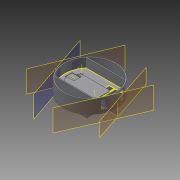
# Autodesk Inventor part: base
Saved by Autodesk Inventor 2014 (Build 180170000, 170)
## iProperties
Created: 2013-06-26
Part Number: base
Material: Generisch
Document SubType Name: Modeling
Designer: hanse
Density: 1 g/cm^3
Appearance: Vorgabe
Author: hanse
Autodesk Inventor part; units mm, degrees
ref_plane "YZ Plane" through (0, 0, 0) normal (1, 0, 0) x (0, 1, 0)
ref_plane "XZ Plane" through (0, 0, 0) normal (0, 1, 0) x (-1, 0, 0)
ref_plane "XY Plane" through (0, 0, 0) normal (0, 0, 1) x (1, 0, 0)
sketch "Skizze1" plane through (0, 0, 0) normal (0, 0, 1) x (1, 0, 0)
  line L0 (29, -20.75) -> (-29, -20.75) projected
  line L1 (29, 20.75) -> (29, -20.75) projected
  line L2 (-29, 20.75) -> (29, 20.75) projected
  line L3 (-29, -20.75) -> (-29, 20.75) projected
  line L4 (4, 34.75) -> (14, 34.75) projected
  line L5 (40.5, 34.75) -> (14, 34.75) projected
  line L6 (14, -34.75) -> (40.5, -34.75) projected
  line L7 (14, -34.75) -> (4, -34.75) projected
  line L8 (40.5, -34.75) -> (40.5, -21.05) projected
  line L9 (40.5, -21.05) -> (40.5, -7.75) projected
  line L10 (40.5, 21.05) -> (40.5, 7.75) projected
  line L11 (40.5, 34.75) -> (40.5, 21.05) projected
  line L12 (4, 34.75) -> (4, 21.05)
  line L13 (4, -34.75) -> (4, -21.05)
  line L14 (13.5, 17.844) -> (13.5, 38.186)
  line L15 (13.5, -17.844) -> (13.5, -38.186)
  line L16 (0, 0) -> (29, 0)
  line L17 (13.5, 17.844) -> (13.5, -17.844)
  line L18 (-15.5, 46.05) -> (42.5, 46.05) projected
  line L19 (42.5, 38.05) -> (-15.5, 38.05) projected
  line L20 (-15.5, -38.05) -> (42.5, -38.05) projected
  line L21 (42.5, -46.05) -> (-15.5, -46.05) projected
  circle A0 centre (12.6975, 0) radius 58.0715
  line L22 (40.5, -7.75) -> (29, -7.75)
  line L23 (29, -7.75) -> (29, -26.5586)
  line L24 (29, -26.5586) -> (40.5, -26.5586)
  line L25 (40.5, -26.5586) -> (40.5, -7.75)
  line L26 (40.5, 7.75) -> (40.5, 26.6995)
  line L27 (40.5, 26.6995) -> (29, 26.6995)
  line L28 (29, 26.6995) -> (29, 7.75)
  line L29 (40.5, 7.75) -> (38.25, 7.75) projected
  line L30 (38.25, 7.75) -> (31.25, 7.75) projected
  line L31 (31.25, 7.75) -> (29, 7.75) projected
  line L32 (40.5, 7.75) -> (29, 7.75)
  line L33 (-32.2663, 36.75) -> (57.6613, 36.75)
  line L34 (-32.2663, -36.75) -> (57.6613, -36.75)
  line L35 (66.1683, 16.4065) -> (68.2, 17.0815)
  dimension "d0" = 2
  dimension "d1" = 2
  constraints: 34 end point, 5 parallel, 5 point on circle, 4 point on line, 4 vertical, 3 collinear, 2 perpendicular, 1 centre point, 1 horizontal, 1 midpoint, 6 other
  measures "d0" distance between parallel lines of L5 L33
  measures "d1" distance between parallel lines of L6 L34
ref_plane "Arbeitsebene1" through (30, 21.05, 2.35) normal (0, 0, 1) x (1, 0, 0)
extrude "Extrusion1" add sketch "Skizze1" along normal up to surface (2.35 mm away) contours L23 L24 L8 L6 L7 L15 L0 | L0 L15 L17 L16 L1 | L15 L34 A0 L33 L14 L2 L3 L0 | L0 L3 L2 L14 L17 L15 | L1 L31 L30 L29 L10 L11 L5 L4 L14 L33 A0 L34 L15 L7 L6 L8 L9 L22 | L16 L17 L14 L2 L1 | L14 L4 L5 L11 L27 L28 L2
sketch "Skizze2" plane through (0, 0, 0) normal (0, 0, -1) x (-1, 0, 0)
  line L0 (-29, 26.6995) -> (-29, 7.75) projected
  line L1 (-29, 7.75) -> (-40.5, 7.75) projected
  line L2 (-40.5, 7.75) -> (-40.5, 26.6995) projected
  line L3 (-40.5, 26.6995) -> (-29, 26.6995) projected
  line L4 (-40.5, -26.5586) -> (-40.5, -7.75) projected
  line L5 (-40.5, -7.75) -> (-29, -7.75) projected
  line L6 (-29, -7.75) -> (-29, -26.5586) projected
  line L7 (-29, -26.5586) -> (-40.5, -26.5586) projected
  line L8 (-57.6613, 36.75) -> (32.2663, 36.75) projected
  line L9 (32.2663, -36.75) -> (-57.6613, -36.75) projected
  line L10 (-29, -20.75) -> (29, -20.75) projected
  line L11 (29, 20.75) -> (-29, 20.75) projected
  line L12 (-42.5, 36.75) -> (-42.5, -36.75)
  line L13 (-29, 7.75) -> (-29, -7.75)
  line L14 (1, 36.75) -> (1, 20.75)
  line L15 (1, -20.75) -> (1, -36.75)
  line L16 (-4, 34.75) -> (-4, 21.05)
  line L17 (-4, -34.75) -> (-4, -21.05)
  point P0 (0, 0)
  dimension "d4" = 2
  dimension "d5" = 5
  constraints: 12 end point, 6 point on line, 3 perpendicular, 2 collinear, 2 vertical, 4 other
  measures "d4" distance between parallel lines of L2 L12
  measures "d5" distance between parallel lines of L14 L16
ref_plane "Arbeitsebene2" through (14, 21.05, -20) normal (0, 0, -1) x (0, 1, 0)
extrude "Extrusion2" add sketch "Skizze2" along normal up to surface (20 mm away) contours L3 L2 L1 L13 L5 L4 L7 L6 L10 L15 L9 L12 L8 L14 L11 L0
sketch "Skizze3" plane through (-1, 20.75, 0) normal (0, -1, 0) x (1, 0, 0)
  line L0 (0, -20) -> (30, -20) projected
  line L1 (30, 0) -> (30, -20) projected
  line L2 (0, 0) -> (30, 0) projected
  line L3 (30, -20) -> (41.5, -20) projected
  line L4 (41.5, -20) -> (30, -20)
  line L5 (30, -20) -> (30, 0)
  line L6 (30, 0) -> (41.5, 0)
  line L7 (41.5, 0) -> (41.5, -20)
  arc A0 (15, 0) -> (15, -20) centre (15, -10) ccw projected
  point P0 (1, 0)
  constraints: 8 end point, 2 parallel, 1 horizontal, 1 perpendicular
ref_plane "Arbeitsebene3" through (4, 34.75, -20) normal (0, 1, 0) x (0, 0, 1)
extrude "Extrusion3" cut sketch "Skizze3" against normal up to surface (14 mm away) contours L1 L6 L7 L3
sketch "Skizze4" plane through (14, 34.75, 0) normal (0, -1, 0) x (1, 0, 0)
  circle A0 centre (8.9, -11.9) radius 1.5 projected
  circle A1 centre (-0.5, -10) radius 2.5 projected
  circle A2 centre (15.5, -6.5) radius 1.5 projected
  point P0 (-14, 0)
extrude "Extrusion4" cut sketch "Skizze4" against normal blind 0.5
ref_plane "Arbeitsebene13" through (0, 0, 0) normal (0, 1, 0) x (1, 0, 0)
sketch "Skizze5" plane through (14, 34.75, -20) normal (0, -1, 0) x (1, 0, 0)
  circle A0 centre (-0.5, 10) radius 1.5 projected
  point P0 (-14, 20)
extrude "Extrusion5" cut sketch "Skizze5" against normal through all
mirror "Spiegeln1" about plane through (0, 0, 0) normal (0, 1, 0) of "Extrusion5", "Extrusion3"
sketch "Skizze6" plane through (14, -34.75, 0) normal (0, 1, 0) x (1, 0, 0)
  circle A0 centre (15.5, 13.5) radius 1.5 projected
  circle A1 centre (8.9, 8.1) radius 1.5 projected
  circle A2 centre (-0.5, 10) radius 2.5 projected
  point P0 (-14, 0)
extrude "Extrusion6" cut sketch "Skizze6" against normal blind 0.5
sketch "Skizze7" plane through (42.5, 36.75, -20) normal (0, 0, -1) x (-1, 0, 0)
  line L0 (43.5, -73.5) -> (0, -73.5)
  line L1 (0, -73.5) -> (0, 0)
  line L2 (0, 0) -> (43.5, 0)
  line L3 (43.5, 0) -> (43.5, -73.5)
  point P0 (42.5, -36.75)
  constraints: 8 end point, 2 parallel, 1 horizontal, 1 perpendicular
extrude "Extrusion7" add sketch "Skizze7" along normal blind 2
sketch "Skizze8" plane through (42.5, 36.75, -22) normal (0, 0, -1) x (-1, 0, 0)
  line L0 (43.5, -73.5) -> (43.5, 0) projected
  line L1 (71.5, -16) -> (13.5, -16) projected
  line L2 (13.5, -57.5) -> (71.5, -57.5) projected
  line L3 (13.5, -16) -> (43.5, -16)
  line L4 (43.5, -16) -> (43.5, -57.5)
  line L5 (43.5, -57.5) -> (13.5, -57.5)
  line L6 (13.5, -57.5) -> (13.5, -16)
  line L7 (11.25, -12.5) -> (11.25, -29) projected
  line L8 (4.25, -29) -> (11.25, -29) projected
  line L9 (4.25, -12.5) -> (4.25, -29) projected
  line L10 (11.25, -12.5) -> (4.25, -12.5) projected
  line L11 (11.25, -61) -> (4.25, -61) projected
  line L12 (4.25, -61) -> (4.25, -44.5) projected
  line L13 (11.25, -44.5) -> (4.25, -44.5) projected
  line L14 (11.25, -61) -> (11.25, -44.5) projected
  line L15 (13.5, -44.5) -> (13.5, -63.3086) projected
  line L16 (13.5, -63.3086) -> (2, -63.3086) projected
  line L17 (2, -63.3086) -> (2, -44.5) projected
  line L18 (2, -44.5) -> (13.5, -44.5) projected
  line L19 (2, -10.0505) -> (13.5, -10.0505) projected
  line L20 (13.5, -10.0505) -> (13.5, -29) projected
  line L21 (13.5, -29) -> (2, -29) projected
  line L22 (2, -29) -> (2, -10.0505) projected
  point P0 (42.5, -36.75)
  constraints: 8 end point, 2 parallel, 2 point on line, 1 horizontal, 1 perpendicular
extrude "Extrusion8" cut sketch "Skizze8" against normal up to next
fillet "Rundung1" radius 17 2 edges at (-1, 28.75, -22) (-1, -28.75, -22)
sketch "Skizze25" plane through (-1, 20.75, 0) normal (0, -1, 0) x (1, 0, 0)
  line L0 (30, 0) -> (30, -22) projected
  line L1 (0, 0) -> (30, 0) projected
  arc A0 (15, 0) -> (15, -20) centre (15, -10) ccw projected
  line L2 (15, -20) -> (31, -20) projected
  line L3 (31, 0) -> (15, 0) projected
  circle A1 centre (15, -10) radius 10
  line L4 (15, -20) -> (30, -20)
  line L5 (30, -20) -> (30, 0)
  line L6 (30, 0) -> (15, 0)
  point P0 (1, 0)
  constraints: 6 end point, 2 collinear, 2 point on line, 2 tangent, 1 centre point, 1 coincident, 1 concentric
ref_plane "Arbeitsebene12" through (4, 34.75, -20) normal (0, 1, 0) x (0, 0, 1)
extrude "Extrusion25" cut sketch "Skizze25" against normal up to surface (14 mm away)
sketch "Skizze26" plane through (29, 20.75, -22) normal (0, -1, 0) x (1, 0, 0)
  line L0 (0, 2) -> (0, 0) projected
  line L1 (0, 2) -> (-15, 2) projected
  line L2 (-13, 0) -> (0, 0)
  line L3 (0, 0) -> (0, 3.5)
  line L4 (0, 3.5) -> (-13, 3.5)
  line L5 (-13, 3.5) -> (-13, 0)
  point P0 (-29, 22)
  dimension "d166" = 1.5
  constraints: 8 end point, 2 parallel, 1 collinear, 1 horizontal, 1 perpendicular
  measures "d166" distance between parallel lines of L1 L4
extrude "Extrusion26" add sketch "Skizze26" along normal blind 1.5
sketch "Skizze27" plane through (16, 20.75, -20) normal (-1, 0, 0) x (0, 0, 1)
  line L0 (1.5, 0) -> (0, 0) projected
  line L1 (1.5, -1.5) -> (-2, -1.5) projected
  line L2 (1.5, 0) -> (1.5, -1.5) projected
  line L3 (0, 0) -> (1.5, -0.546)
  line L4 (0, -1.5) -> (1.5, -0.634)
  point P0 (20, -20.75)
  dimension "d169" = 30
  dimension "d170" = 20
  constraints: 4 end point, 3 point on line
  measures "d169" angle of L1 L4
  measures "d170" angle of L0 L3
extrude "Extrusion27" cut sketch "Skizze27" against normal up to next
mirror "Spiegeln3" about plane through (0, 0, 0) normal (0, 1, 0) of "Extrusion25", "Extrusion26", "Extrusion27"
sketch "Skizze9" plane through (-32.2663, 36.75, 2.35) normal (0, 0, 1) x (1, 0, 0)
  line L0 (0, 0) -> (89.9275, 0) projected
  line L1 (89.9275, -73.5) -> (0, -73.5) projected
  arc A0 (89.9275, -73.5) -> (89.9275, 0) centre (44.9638, -36.75) ccw projected
  arc A1 (0, 0) -> (0, -73.5) centre (44.9638, -36.75) ccw projected
  circle A2 centre (44.9638, -36.75) radius 58.0715
  circle A3 centre (44.9638, -36.75) radius 56.0715
  line L2 (0.9586, -2) -> (88.9689, -2)
  line L3 (0.9586, -71.5) -> (88.9689, -71.5)
  line L4 (2.6146, -73.5) -> (87.3129, -73.5)
  line L5 (2.6146, 0) -> (87.3129, 0)
  point P0 (32.2663, -36.75)
  point P1 (0, -2)
  dimension "d174" = 2
  dimension "d175" = 2
  dimension "d176" = 2
  constraints: 8 end point, 4 point on circle, 4 point on line, 2 coincident, 2 parallel, 1 centre point, 1 concentric, 10 other
  measures "d175" distance between parallel lines of L0 L2
  measures "d176" distance between parallel lines of L3 L1
extrude "Extrusion9" add sketch "Skizze9" along normal blind 20 contours A2 L0 A3 | L0 A3 L1 A1 | L0 A3 L2 | L1 A3 A2 | A0 L1 A3 L0 | A3 L3 L1
sketch "Skizze28" plane through (-31.3076, -34.75, 2.35) normal (0, 0, 1) x (1, 0, 0)
  line L0 (0, 0) -> (88.0103, 0) projected
  arc A0 (88.0103, 0) -> (88.0103, 69.5) centre (44.0052, 34.75) ccw projected
  line L1 (88.0103, 69.5) -> (0, 69.5) projected
  arc A1 (0, 69.5) -> (0, 0) centre (44.0052, 34.75) ccw projected
  line L2 (73.8076, -2) -> (73.8076, 71.5) projected
  line L3 (73.8076, 69.5) -> (73.8076, 0)
  line L4 (73.8076, 0) -> (88.0103, 0)
  line L5 (73.8076, 69.5) -> (88.0103, 69.5)
  circle A2 centre (44.0052, 34.75) radius 56.0715
  line L6 (73.8076, 61.5) -> (93.2845, 61.5)
  line L7 (73.8076, 8) -> (93.2845, 8)
  point P0 (31.3076, 34.75)
  dimension "d187" = 8
  dimension "d188" = 8
  constraints: 10 end point, 6 point on line, 5 point on circle, 2 collinear, 2 perpendicular, 1 centre point, 1 coincident
  measures "d187" distance between parallel lines of L1 L6
  measures "d188" distance between parallel lines of L4 L7
extrude "Extrusion28" cut sketch "Skizze28" against normal up to next contours L2 L6 A0 L7
sketch "Skizze29" plane through (42.5, 36.75, -22) normal (0, 0, -1) x (-1, 0, 0)
  line L0 (0, 0) -> (0, -73.5) projected
  line L1 (2, -44.5) -> (13.5, -44.5) projected
  line L2 (13.5, -44.5) -> (13.5, -29) projected
  line L3 (13.5, -29) -> (2, -29) projected
  line L4 (2, -29) -> (0, -29)
  line L5 (2, -44.5) -> (0, -44.5)
  point P0 (42.5, -36.75)
  point P1 (0, -2)
  point P2 (0, -71.5)
  constraints: 4 end point, 2 perpendicular, 2 point on line
extrude "Extrusion29" cut sketch "Skizze29" against normal up to surface (22 mm away)
sketch "Skizze30" plane through (0, 0, 0) normal (0, 0, -1) x (-1, 0, 0)
  line L0 (-29, 26.6995) -> (-29, 7.75) projected
  line L1 (-42.5, 7.75) -> (-29, 7.75)
  line L2 (-29, 7.75) -> (-29, 5.75)
  line L3 (-29, 5.75) -> (-42.5, 5.75)
  line L4 (-42.5, 5.75) -> (-42.5, 7.75)
  point P0 (0, 0)
  dimension "d181" = 2
  constraints: 8 end point, 2 parallel, 1 collinear, 1 horizontal, 1 perpendicular
  measures "d181" distance between parallel lines of L3 L1
extrude "Extrusion30" add sketch "Skizze30" along normal blind 1.5
chamfer "Fase1" distance 2 distance2 1.5 1 edges at (35.75, 5.75, -1.5) measured on face at (35.75, 6.25, -1.5)
mirror "Spiegeln4" about plane through (0, 0, 0) normal (0, 1, 0) of "Extrusion30", "Fase1"
sketch "Skizze31" plane through (-31.3076, 34.75, 2.35) normal (0, 0, 1) x (1, 0, 0)
  line L0 (71.8076, -42.5) -> (60.3076, -42.5) projected
  line L1 (71.8076, -61.3086) -> (71.8076, -42.5) projected
  line L2 (60.3076, -61.3086) -> (71.8076, -61.3086) projected
  line L3 (60.3076, -42.5) -> (60.3076, -61.3086) projected
  line L4 (60.3076, -8.0505) -> (60.3076, -27) projected
  line L5 (71.8076, -8.0505) -> (60.3076, -8.0505) projected
  line L6 (71.8076, -27) -> (71.8076, -8.0505) projected
  line L7 (60.3076, -27) -> (71.8076, -27) projected
  line L8 (93.2845, -61.5) -> (73.8076, -61.5) projected
  line L9 (73.8076, -61.5) -> (73.8076, -8) projected
  line L10 (73.8076, -8) -> (93.2845, -8) projected
  arc A0 (93.2845, -8) -> (88.0103, 0) centre (44.0052, -34.75) ccw projected
  line L11 (88.0103, 0) -> (0, 0) projected
  arc A1 (0, 0) -> (0, -69.5) centre (44.0052, -34.75) ccw projected
  line L12 (0, -69.5) -> (88.0103, -69.5) projected
  arc A2 (88.0103, -69.5) -> (93.2845, -61.5) centre (44.0052, -34.75) ccw projected
  point P0 (31.3076, -34.75)
  point P1 (63.8028, -45.1094)
  point P2 (9.3213, -19.5701)
  constraints: 2 other
sketch "Skizze32" plane through (-31.3076, 34.75, 2.35) normal (0, 0, 1) x (1, 0, 0)
  line L0 (71.8076, -42.5) -> (60.3076, -42.5) projected
  circle A0 centre (9.3213, -19.5701) radius 2.5
  line L1 (18.1349, -38.545) -> (64.8001, -38.545) construction
  line L2 (18.1349, -58.3903) -> (64.8001, -58.3903)
  line L3 (64.8001, -18.6996) -> (18.1349, -18.6996)
  arc A1 (18.1349, -18.6996) -> (18.1349, -58.3903) centre (18.1349, -38.545) ccw
  arc A2 (64.8001, -58.3903) -> (64.8001, -18.6996) centre (64.8001, -38.545) ccw
  line L4 (73.8076, -61.5) -> (73.8076, -8) projected
  line L5 (73.8076, -20.8616) -> (73.8076, -56.2283)
  point P0 (31.3076, -34.75)
  point P1 (41.4675, -38.545)
  dimension "d189" = 5
  constraints: 10 end point, 6 point on circle, 4 tangent, 3 centre point, 2 parallel, 2 point on line, 1 coincident, 1 midpoint
  measures "d189" diameter of A0
extrude "Extrusion31" add sketch "Skizze32" along normal blind 2 contours A0 A1 | A1 A0 | A0 A1 L3 A2 L4 L2
sketch "Skizze39" plane through (-32.2663, 36.75, 2.35) normal (0, 0, -1) x (-1, 0, 0)
  arc A0 (-89.9275, -73.5) -> (0, -73.5) centre (-44.9638, -36.75) ccw projected
  arc A1 (-87.3129, -73.5) -> (-2.6146, -73.5) centre (-44.9638, -36.75) ccw projected
  circle A2 centre (-44.9638, -36.75) radius 56.0715
  circle A3 centre (-44.9638, -36.75) radius 58.0715
  point P0 (-32.2663, -36.75)
  constraints: 2 centre point, 2 coincident, 2 concentric
extrude "Extrusion38" add sketch "Skizze39" along normal blind 10
sketch "Skizze33" plane through (-31.3076, 34.75, 4.35) normal (0, 0, 1) x (1, 0, 0)
  line L0 (-5.908, -24.3598) -> (14.292, -24.3744)
  line L1 (14.292, -24.3744) -> (14.2804, -40.5744)
  line L2 (14.2804, -40.5744) -> (-5.9196, -40.5598)
  line L3 (-5.9196, -40.5598) -> (-5.908, -24.3598)
  line L4 (12.7814, -39.0733) -> (-4.4186, -39.0609) projected
  line L5 (-4.4186, -39.0609) -> (-4.409, -25.8609) projected
  line L6 (-4.409, -25.8609) -> (12.791, -25.8733) projected
  line L7 (12.791, -25.8733) -> (12.7814, -39.0733) projected
  point P0 (31.3076, -34.75)
  constraints: 8 end point
extrude "Extrusion32" cut sketch "Skizze33" against normal blind 3 contours L0 L1 L2 L3 | L4 L5 L6 L7
sketch "Skizze34" plane through (-31.3076, 34.75, 4.35) normal (0, 0, 1) x (1, 0, 0)
  arc A0 (11.816, -19.7325) -> (7.8361, -21.5811) centre (9.3213, -19.5701) ccw projected
  circle A1 centre (9.3213, -19.5701) radius 1.45
  point P0 (31.3076, -34.75)
  dimension "d198" = 2.9
  constraints: 1 centre point, 1 coincident
  measures "d198" diameter of A1
extrude "Extrusion33" cut sketch "Skizze34" against normal up to next
ref_plane "Arbeitsebene16" through (67.8071, 18.3094, 0) normal (0.9489949, 0.3152913, 0) x (-0.3152913, 0.9489949, 0)
ref_plane "Arbeitsebene15" through (66.7724, 16.4065, 9.1734) normal (0.9489949, 0.3152913, 0) x (0.3152913, -0.9489949, 0)
sketch "Skizze35" plane through (67.8071, 18.3094, 0) normal (0.9489949, 0.3152913, 0) x (-0.3152913, 0.9489949, 0)
  line L0 (4.8879, 18.8484) -> (-7.8471, 18.8484) projected
  line L1 (4.8879, -0.5016) -> (4.8879, 18.8484) projected
  line L2 (-7.8471, 18.8484) -> (-7.8471, -0.5016) projected
  line L3 (-7.8471, -0.5016) -> (4.8879, -0.5016) projected
  point P0 (4.0034, 0)
extrude "Extrusion34" cut sketch "Skizze35" against normal up to surface round surface about axis through (12.6975, 0, 2.35) along (0, 0, -1) radius 56.0715 far side no
ref_plane "Arbeitsebene18" through (65.9031, -23.2694, 0) normal (0.9162079, -0.4007033, 0) x (0.4007033, 0.9162079, 0)
ref_plane "Arbeitsebene17" through (65.0155, -20.5414, 9.1734) normal (0.9162079, -0.4007033, 0) x (-0.4007033, -0.9162079, 0)
sketch "Skizze36" plane through (65.9031, -23.2694, 0) normal (0.9162079, -0.4007033, 0) x (0.4007033, 0.9162079, 0)
  line L0 (8.5113, 18.8484) -> (-4.2237, 18.8484) projected
  line L1 (8.5113, -0.5016) -> (8.5113, 18.8484) projected
  line L2 (-4.2237, 18.8484) -> (-4.2237, -0.5016) projected
  line L3 (-4.2237, -0.5016) -> (8.5113, -0.5016) projected
  point P0 (-5.0879, 0)
extrude "Extrusion35" cut sketch "Skizze36" against normal up to surface round surface about axis through (12.6975, 0, 2.35) along (0, 0, -1) radius 56.0715 far side no
ref_plane "Arbeitsebene20" through (-41.0608, 21.9623, 0) normal (0.9257263, -0.3781942, 0) x (0.3781942, 0.9257263, 0)
ref_plane "Arbeitsebene19" through (-37.2052, 20.5059, 9.1734) normal (0.9257263, -0.3781942, 0) x (-0.3781942, -0.9257263, 0)
sketch "Skizze37" plane through (-41.0608, 21.9623, 0) normal (0.9257263, -0.3781942, 0) x (0.3781942, 0.9257263, 0)
  line L0 (6.4775, 18.8484) -> (-6.2575, 18.8484) projected
  line L1 (-6.2575, -0.5016) -> (6.4775, -0.5016) projected
  line L2 (6.4775, -0.5016) -> (6.4775, 18.8484) projected
  line L3 (-6.2575, 18.8484) -> (-6.2575, -0.5016) projected
  point P0 (-4.8021, 0)
extrude "Extrusion36" cut sketch "Skizze37" along normal up to surface round surface about axis through (12.6975, 0, 2.35) along (0, 0, -1) radius 56.0715 far side no
ref_plane "Arbeitsebene22" through (-42.3479, -18.5014, 0) normal (-0.9478901, -0.3185975, 0) x (0.3185975, -0.9478901, 0)
ref_plane "Arbeitsebene21" through (-40.3318, -16.041, 9.1734) normal (-0.9478901, -0.3185975, 0) x (-0.3185975, 0.9478901, 0)
sketch "Skizze38" plane through (-42.3479, -18.5014, 0) normal (-0.9478901, -0.3185975, 0) x (0.3185975, -0.9478901, 0)
  line L0 (-8.0574, 18.8484) -> (4.6776, 18.8484) projected
  line L1 (4.6776, -0.5016) -> (-8.0574, -0.5016) projected
  line L2 (-8.0574, -0.5016) -> (-8.0574, 18.8484) projected
  line L3 (4.6776, 18.8484) -> (4.6776, -0.5016) projected
  point P0 (-4.0454, 0)
extrude "Extrusion37" cut sketch "Skizze38" against normal up to surface round surface about axis through (12.6975, 0, 2.35) along (0, 0, -1) radius 56.0715 far side no
ref_plane "Arbeitsebene24" through (-45.374, 0.0419, 0) normal (-0.9999997, 0.0007216, 0) x (-0.0007216, -0.9999997, 0)
ref_plane "Arbeitsebene23" through (-35.7262, -4.3109, 19.15) normal (-0.9999997, 0.0007216, 0) x (0, 0, 1)
sketch "Skizze40" plane through (-45.374, 0.0419, 0) normal (-0.9999997, 0.0007216, 0) x (-0.0007216, -0.9999997, 0)
  line L0 (-8.8541, 19.15) -> (4.3459, 19.15) projected
  line L1 (-8.8541, 19.15) -> (-8.8541, 3.15) projected
  line L2 (4.3459, 3.15) -> (-8.8541, 3.15) projected
  line L3 (4.3459, 19.15) -> (4.3459, 3.15) projected
  point P0 (0.0092, 0)
extrude "Extrusion39" cut sketch "Skizze40" against normal up to surface round surface about axis through (12.6975, 0, 2.35) along (0, 0, -1) radius 56.0715 far side no
sketch "Skizze11" plane through (-32.2663, 36.75, 22.35) normal (0, 0, 1) x (1, 0, 0)
  line L0 (0, -2) -> (81.8398, -2) projected
  line L1 (81.8398, -2) -> (81.8398, -3.0667) projected
  arc A0 (81.8398, -70.4333) -> (81.8398, -3.0667) centre (40.9199, -36.75) ccw projected
  line L2 (81.8398, -70.4333) -> (81.8398, -71.5) projected
  line L3 (81.8398, -71.5) -> (0, -71.5) projected
  line L4 (0, -71.5) -> (0, -70.4333) projected
  arc A1 (0, -3.0667) -> (0, -70.4333) centre (40.9199, -36.75) ccw projected
  line L5 (0, -3.0667) -> (0, -2) projected
  arc A2 (0, 0) -> (0, -73.5) centre (40.9199, -36.75) ccw projected
  line L6 (0, -73.5) -> (81.8398, -73.5) projected
  arc A3 (81.8398, -73.5) -> (81.8398, 0) centre (40.9199, -36.75) ccw projected
  line L7 (81.8398, 0) -> (0, 0) projected
  circle A4 centre (40.9199, -36.75) radius 53
  circle A5 centre (40.9199, -36.75) radius 55
  line L8 (15.0762, 11.8) -> (66.7636, 11.8) projected
  line L9 (66.7636, -85.3) -> (15.0762, -85.3) projected
  line L10 (19.662, 11.8) -> (62.1778, 11.8)
  line L11 (62.1778, -85.3) -> (19.662, -85.3)
  point P0 (32.2663, -36.75)
  constraints: 5 point on circle, 4 end point, 4 point on line, 2 coincident, 1 centre point, 3 other
sketch "Skizze23" plane through (-32.2663, 36.75, 22.35) normal (0, 0, 1) x (1, 0, 0)
  arc A0 (19.662, -85.3) -> (62.1778, -85.3) centre (40.9199, -36.75) ccw projected
  line L0 (62.1778, -85.3) -> (19.662, -85.3) projected
  arc A1 (62.1778, 11.8) -> (19.662, 11.8) centre (40.9199, -36.75) ccw projected
  line L1 (19.662, 11.8) -> (62.1778, 11.8) projected
  point P0 (32.2663, -36.75)
sketch "Skizze12" plane through (13.5, 0, 17.35) normal (0, 0, 1) x (1, 0, 0)
  line L0 (-38.1895, 36.75) -> (38.1895, 36.75) projected
  line L1 (40.9199, -34.75) -> (-40.9199, -34.75) projected
  line L2 (-40.9199, -34.75) -> (-40.9199, -33.6833) projected
  arc A0 (-40.9199, 33.6833) -> (-40.9199, -33.6833) centre (0, 0) ccw projected
  line L3 (-40.9199, 33.6833) -> (-40.9199, 34.75) projected
  line L4 (-40.9199, 34.75) -> (40.9199, 34.75) projected
  line L5 (40.9199, 34.75) -> (40.9199, 33.6833) projected
  arc A1 (40.9199, -33.6833) -> (40.9199, 33.6833) centre (0, 0) ccw projected
  line L6 (40.9199, -33.6833) -> (40.9199, -34.75) projected
  line L7 (-15.9199, 34.75) -> (-15.9199, 36.75)
  line L8 (-15.9199, 36.75) -> (-10.9199, 36.75)
  line L9 (-10.9199, 36.75) -> (-10.9199, 34.75)
  line L10 (-10.9199, 34.75) -> (-15.9199, 34.75)
  line L11 (15.9199, 36.75) -> (10.9199, 36.75)
  line L12 (10.9199, 36.75) -> (10.9199, 34.75)
  line L13 (15.9199, 34.75) -> (10.9199, 34.75)
  line L14 (15.9199, 34.75) -> (15.9199, 36.75)
  point P0 (-13.5, 0)
  dimension "d158" = 25
  dimension "d159" = 25
  dimension "d160" = 5
  dimension "d161" = 5
  constraints: 16 end point, 8 point on line, 4 perpendicular, 2 collinear
  measures "d158" distance between parallel lines of L7 L3
  measures "d159" distance between parallel lines of L14 L5
  measures "d160" distance of L9.end L7.start
  measures "d161" distance of L11.start L11.end
